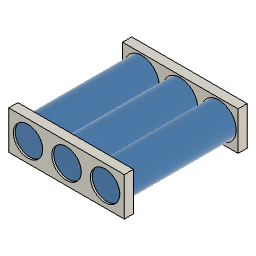
BatteryPack v23 (Autodesk Fusion 360 design; units mm, degrees)
Autodesk Fusion 360 part; units mm, degrees
sketch "Sketch2" plane through (0, 0, 0) normal (0, 1, 0) x (1, 0, 0) in component "Battery"
  circle A0 centre (0, 0) radius 9
  dimension "d91" = 18
  constraint coincident A0.centre origin
  measures "d91" diameter of A0
extrude "Extrude2" add sketch "Sketch2" along normal blind 65 makes body 1 in component "Battery"
sketch "Sketch2 (2)" plane through (0, 0, 0) normal (0, -1, 0) x (1, 0, 0) in component "Holder"
  circle A0 centre (0, 0) radius 9 construction
  circle A1 centre (0, 0) radius 9.5
  circle A2 centre (0, 0) radius 10.5
  circle A3 centre (0, 0) radius 8
  line L0 (10.5, 10.5) -> (10.5, -10.5) construction
  line L1 (10.5, -10.5) -> (0, -10.5)
  line L2 (10.5, 10.5) -> (0, 10.5)
  circle A4 centre (21, 0) radius 10.5
  circle A5 centre (21, 0) radius 9.5
  circle A6 centre (21, 0) radius 8
  line L3 (10.5, 10.5) -> (21, 10.5)
  line L4 (10.5, -10.5) -> (21, -10.5)
  line L5 (31.5, 10.5) -> (31.5, -10.5) construction
  circle A7 centre (42, 0) radius 10.5
  circle A8 centre (42, 0) radius 9.5
  circle A9 centre (42, 0) radius 8
  line L6 (52.5, -10.5) -> (-10.5, -10.5)
  line L7 (-10.5, -10.5) -> (-10.5, 10.5)
  line L8 (-10.5, 10.5) -> (52.5, 10.5)
  line L9 (52.5, 10.5) -> (52.5, -10.5)
  line L10 (52.5, -10.5) -> (-10.5, 10.5) construction
  line L11 (-10.5, -10.5) -> (52.5, 10.5) construction
  circle A10 centre (21, 0) radius 9 construction
  circle A11 centre (42, 0) radius 9 construction
  point P0 (21, 0)
  dimension "d94" = 0.5
  dimension "d95" = 1.5
  dimension "d96" = -1
  constraint vertical L0
  constraint coincident A2 L1.end
  constraint coincident A2 L2.end
  constraint perpendicular L0 L2
  constraint perpendicular L0 L1
  constraint tangent A2 L2
  constraint tangent A2 L1
  constraint tangent A2 L0
  constraint symmetric A1 L0 A5
  constraint symmetric A2 L0 A4
  constraint symmetric A3 L0 A6
  constraint symmetric L2.start L0 L3.start
  constraint symmetric L1.start L0 L4.start
  constraint symmetric L0 L1.end L4.end
  constraint symmetric L0 L2.end L3.end
  constraint vertical L5
  constraint tangent A4 L5
  constraint symmetric A4 L5 A7
  constraint symmetric A5 L5 A8
  constraint symmetric A6 L5 A9
  constraint horizontal L6
  constraint perpendicular L6 L7
  constraint parallel L6 L8
  constraint parallel L7 L9
  constraint coincident L10 P0
  constraint coincident L11 P0
  constraint coincident P0 A4.centre
  constraint tangent A2 L8
  constraint tangent A2 L7
  constraint coincident L5.end L6
  constraint coincident L5.start L8
  constraint symmetric A0 L0 A10
  constraint symmetric L5 A10 A11
extrude "Extrude1" add sketch "Sketch2 (2)" against normal blind 4 separate body contours A2 | A2 L1 A4 L4 L6 | A2 L2 A4 L3 L8 | A4 | A2 L7 L8 | A2 L6 L7 | A4 A7 L8 | A4 A7 L6 | A7 | A7 L8 L9 | A7 L6 L9 makes body 2 in component "Holder"
extrude "Extrude2'" add sketch "Sketch2 (2)" along normal blind 1 contours A1 | A2 | A2 L1 A4 L4 L6 | A2 L2 A4 L3 L8 | A4 | A2 L7 L8 | A2 L6 L7 | A4 A7 L8 | A4 A7 L6 | A7 | A7 L8 L9 | A7 L6 L9 | A5 | A8 bodies 2 in component "Holder"
component "Battery" placed x (1, 0, 0) y (0, 1, 0) z (0, 0, 1) at (-21, -34, 92.5)
component "Holder" placed x (1, 0, 0) y (0, 1, 0) z (0, 0, 1) at (-21, -34, 92.5)
component "Battery" placed x (1, 0, 0) y (0, 1, 0) z (0, 0, 1) at (0, -34, 92.5)
component "Battery" placed x (1, 0, 0) y (0, 1, 0) z (0, 0, 1) at (21, -34, 92.5)
component "Holder" placed x (1, 0, 0) y (0, -1, 0) z (0, 0, -1) at (-21, 31, 92.5)
